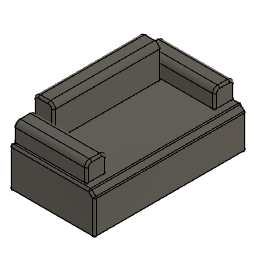
rgiro_yamazen_sofa_double (Autodesk Fusion 360 design; units mm, degrees)
Autodesk Fusion 360 part; units mm, degrees
sketch "Sketch1" plane through (0, 0, 0) normal (0, 0, 1) x (1, 0, 0)
  line L0 (425, -760) -> (-425, -760)
  line L1 (-425, -760) -> (-425, 760)
  line L2 (-425, 760) -> (425, 760)
  line L3 (425, 760) -> (425, -760)
  line L4 (425, -760) -> (-425, 760) construction
  line L5 (-425, -760) -> (425, 760) construction
  line L6 (-405, -740) -> (325, -740)
  line L7 (325, -740) -> (325, -540)
  line L8 (325, -540) -> (-405, -540)
  line L9 (-405, -540) -> (-405, -740)
  line L10 (-405, -540) -> (-205, -540)
  line L11 (-205, -540) -> (-205, 540)
  line L12 (-205, 540) -> (-405, 540)
  line L13 (-405, 540) -> (-405, -540)
  line L14 (-405, 540) -> (325, 540)
  line L15 (325, 540) -> (325, 740)
  line L16 (325, 740) -> (-405, 740)
  line L17 (-405, 740) -> (-405, 540)
  dimension "d1" = 1520
  dimension "d2" = 850
  dimension "d3" = 20
  dimension "d4" = 20
  dimension "d5" = 20
  dimension "d6" = 200
  dimension "d7" = 200
  dimension "d8" = 100
  constraint perpendicular L0 L1
  constraint parallel L0 L2
  constraint parallel L1 L3
  constraint horizontal L0
  constraint coincident L4 origin
  constraint coincident L5 origin
  constraint horizontal L6
  constraint vertical L7
  constraint horizontal L8
  constraint vertical L9
  constraint horizontal L10
  constraint vertical L11
  constraint horizontal L12
  constraint vertical L13
  constraint horizontal L14
  constraint vertical L15
  constraint horizontal L16
  constraint vertical L17
  constraint collinear L9 L13
  constraint collinear L9 L17
  constraint collinear L7 L15
  constraint equal L7 L15
  constraint collinear L8 L10
  constraint collinear L12 L14
  measures "d1" distance of L0.start L2.end
  measures "d2" distance of L0.start L0.end
  measures "d3" distance of L1 L6.start
  measures "d4" distance of L0 L6
  measures "d5" distance of L2 L16
  measures "d6" distance of L6.end L7.end
  measures "d7" distance of L8.end L10.end
  measures "d8" distance of L3 L7
extrude "Extrude1" add sketch "Sketch1" along normal blind 400 contours L0 L1 L2 L3 | L6 L7 L8 L9 L10 | L8 L10 L11 L12 L13 L14 | L12 L14 L15 L16 L17 makes body 1
sketch "Sketch2" plane through (0, 0, 400) normal (0, 0, 1) x (-1, 0, 0)
  line L0 (-425, -760) -> (425, -760)
  line L1 (425, -760) -> (425, 760)
  line L2 (425, 760) -> (-425, 760)
  line L3 (-425, 760) -> (-425, -760)
  line L4 (405, 740) -> (-325, 740)
  line L5 (-325, 540) -> (405, 540)
  line L6 (405, 540) -> (405, 740)
  line L7 (-325, 740) -> (-325, 540)
  line L8 (405, -740) -> (405, -540)
  line L9 (405, -540) -> (-325, -540)
  line L10 (-325, -740) -> (405, -740)
  line L11 (-325, -540) -> (-325, -740)
extrude "Extrude2" add sketch "Sketch2" along normal blind 200 separate body contours L4 L5 L6 L7 | L8 L9 L10 L11 makes body 2 at (81.6667, -540, 466.6667) makes body 3 at (-161.6667, 540, 466.6667)
sketch "Sketch3" plane through (0, 0, 400) normal (0, 0, 1) x (-1, 0, 0)
  line L0 (-425, -760) -> (425, -760)
  line L1 (425, -760) -> (425, 760)
  line L2 (425, 760) -> (-425, 760)
  line L3 (-425, 760) -> (-425, -760)
  line L4 (205, 540) -> (205, -540)
  line L5 (205, -540) -> (405, -540)
  line L6 (405, 540) -> (205, 540)
  line L7 (405, -540) -> (405, 540)
extrude "Extrude3" add sketch "Sketch3" along normal blind 340 separate body contours L4 L5 L6 L7 makes body 4
chamfer "Chamfer2" distance 50 angle 45 1 edges at (425, 0, 400) on bodies 1
fillet "Fillet2" radius 20 7 faces at (425, 253.3333, 116.6667) (391.6667, 253.3333, 383.3333) (125, 760, 133.3333) (-425, -253.3333, 133.3333) (125, -760, 133.3333) (-141.6667, 253.3333, 0) (-158.3333, 253.3333, 400) on bodies 1
fillet "Fillet3" radius 50 6 edges at (-40, -740, 600) (-40, -540, 600) (-40, 540, 600) (-40, 740, 600) (-205, 0, 740) (-405, 0, 740) on bodies 2 3 4
fillet "Fillet4" radius 20 21 faces at (-405, -606.6667, 450) (-161.6667, -740, 450) (-161.6667, -692.3791, 599.9434) (81.6667, -656.6667, 600) (81.6667, -587.6209, 599.9434) (81.6667, -540, 450) (325, -673.3333, 450) (-161.6667, 540, 450) (-161.6667, 585.2472, 599.7736) (81.6667, 623.3333, 600) (81.6667, 692.3791, 599.9434) (81.6667, 740, 450) (325, 606.6667, 450) (-405, 673.3333, 450) (-205, -180, 593.3333) (-220.496, -180, 726.1867) (-288.3333, 180, 740) (-366.7879, 180, 738.5906) (-405, 180, 593.3333) (-271.6667, 540, 496.6667) (-338.3333, -540, 496.6667) on bodies 2 3 4
